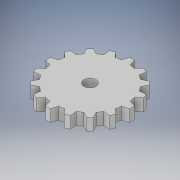
# Autodesk Inventor part: drivenGear
Saved by Autodesk Inventor 2018 (Build 220112000, 112)
## iProperties
Created: 2018-04-19
Part Number: drivenGear
Material: Generic
Document SubType Name: Modeling
Designer: Cole Tucker
Density: 1 g/cm^3
Appearance: Default
Author: Cole Tucker
Autodesk Inventor part; units mm, degrees
ref_plane "YZ Plane" through (0, 0, 0) normal (1, 0, 0) x (0, 1, 0)
ref_plane "XZ Plane" through (0, 0, 0) normal (0, 1, 0) x (-1, 0, 0)
ref_plane "XY Plane" through (0, 0, 0) normal (0, 0, 1) x (1, 0, 0)
sketch "Sketch1" plane through (0, 0, 0) normal (0, 1, 0) x (-1, 0, 0)
  circle A0 centre (0, 0) radius 19.05
  circle A1 centre (0, 0) radius 3.175
  dimension "d0" = 38.1
  dimension "d1" = 6.35
  constraints: 2 centre point, 2 coincident
  measures "d0" diameter of A0
  measures "d1" diameter of A1
extrude "Extrusion1" add sketch "Sketch1" along normal blind 6.35
sketch "Sketch2" plane through (0, 6.35, 0) normal (0, 1, 0) x (1, 0, 0)
  circle A0 centre (0, 0) radius 19.05 projected
  line L0 (0, -19.05) -> (0, -22.225)
  line L1 (0, -22.225) -> (-1.27, -22.225)
  line L2 (0, -22.225) -> (1.27, -22.225)
  line L3 (-2.2961, -18.9111) -> (2.2961, -18.9111)
  line L4 (1.27, -22.225) -> (2.2961, -18.9111)
  line L5 (-2.2961, -18.9111) -> (-1.27, -22.225)
  dimension "d4" = 3.175
  dimension "d5" = 1.27
  dimension "d6" = 1.27
  constraints: 12 end point, 3 point on circle, 2 horizontal, 1 perpendicular, 1 vertical
  measures "d4" distance of L0.start L0.end
  measures "d5" distance of L0.end L1.end
  measures "d6" distance of L0.end L2.end
extrude "Extrusion2" add sketch "Sketch2" against normal blind 6.35 contours A0 L0 L1 L5 | L4 L2 L0 A0
pattern_circular "Circular Pattern1" count 16 over 360 about axis through (0, 0, 0) along (0, 1, 0) of "Extrusion2"
body "Solid1"
